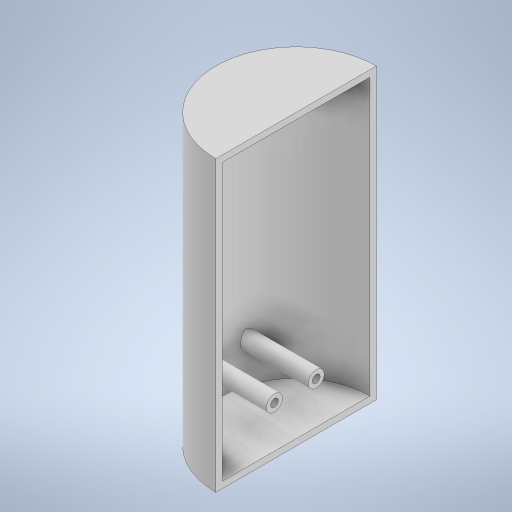
# Autodesk Inventor part: cover2
Saved by Autodesk Inventor 2023 (Build 270158000, 158)
## iProperties
Created: 2023-04-07
Part Number: cover2
Material: Generic
Document SubType Name: Modeling
Designer: user
Density: 1 g/cm^3
Appearance: Default
Author: user
Autodesk Inventor part; units mm, degrees
ref_plane "YZ Plane" through (0, 0, 0) normal (1, 0, 0) x (0, 1, 0)
ref_plane "XZ Plane" through (0, 0, 0) normal (0, 1, 0) x (-1, 0, 0)
ref_plane "XY Plane" through (0, 0, 0) normal (0, 0, 1) x (1, 0, 0)
sketch "Sketch1" plane through (0, 0, 0) normal (1, 0, 0) x (0, 1, 0)
  line L0 (45, 25) -> (-45, 25)
  line L1 (-45, 25) -> (-45, -25)
  line L2 (-45, -25) -> (45, -25)
  line L3 (45, -25) -> (45, 25)
  line L4 (43, -23) -> (-43, -23)
  line L5 (-43, -23) -> (-43, 23)
  line L6 (-43, 23) -> (43, 23)
  line L7 (43, 23) -> (43, -23)
  line L8 (45, 0) -> (-45, 0)
  point P0 (0, 0)
  point P1 (-43, 0)
  point P2 (43, 0)
  dimension "d0" = 2
  dimension "d1" = 90
  dimension "d2" = 45
  dimension "d3" = 50
  dimension "d4" = 25
  constraints: 18 end point, 4 parallel, 2 midpoint, 2 perpendicular, 1 horizontal, 3 other
  measures "d0" distance between parallel lines of L2 L4
  measures "d1" distance between parallel lines of L1 L3
  measures "d2" distance from line of point (0, 0) L1
  measures "d3" distance between parallel lines of L0 L2
  measures "d4" distance from line of point (0, 0) L2
revolve "Revolution1" add sketch "Sketch1" angle 180 about axis through (0, 45, 0) along (0, -1, 0) contours L3 L8 L7 L6 L5 L1 L0
sketch "Sketch2" plane through (0, 0, 0) normal (1, 0, 0) x (0, 1, 0)
  circle A0 centre (-30, 6.75) radius 2.5
  circle A1 centre (-30, 6.75) radius 1.25
  line L0 (-45, 25) -> (-45, -25) projected
  point P0 (0, 0)
  dimension "d7" = 5
  dimension "d10" = 2.5
  dimension "d13" = 6.75
  dimension "d14" = 15
  constraints: 2 centre point, 1 coincident
  measures "d7" diameter of A0
  measures "d10" diameter of A1
  measures "d13" vertical distance of point (0, 0) A0.centre
  measures "d14" distance from line of L0 A0.centre
extrude "Extrusion1" add sketch "Sketch2" against normal up to surface from surface at 0 round surface about axis through (0, 0, 0) along (0, -1, 0) radius 23 far side no
thread "Thread1" size "M2.5x0.45" class "6H" standard "ISO Metric profile" length 20.107
pattern_linear "Rectangular Pattern1" count 2 spacing 13 along (0, 0, -1) of "Extrusion1"
thread "Thread2" size "M2.5x0.45" class "6H" standard "ANSI Metric M Profile" length 20.107
equation "\"d2\" = 0.5 * d1"
equation "\"d4\" = 0.5 * d3"
body "Solid1"
